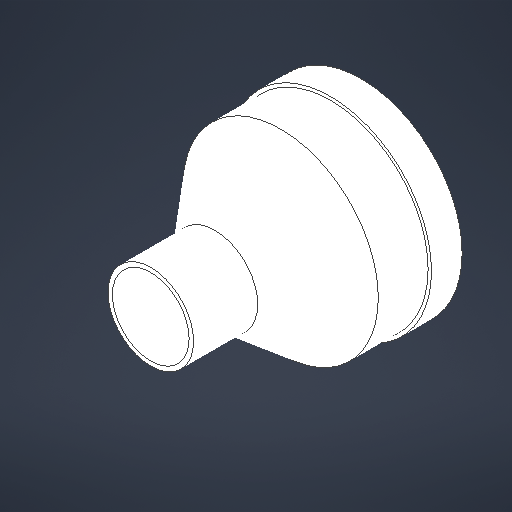
# Autodesk Inventor part: CAPSULA 2DA MITAD
Saved by Autodesk Inventor 2026.2 (Build 302298000, 298)
## iProperties
Created: 2025-12-31
Part Number: CAPSULA 2DA MITAD
Material: Genérico
Document SubType Name: Modeling
Designer: vicho
Density: 1 g/cm^3
Appearance: Valor por defecto
Author: vicho
Autodesk Inventor part; units mm, degrees
ref_plane "YZ Plane" through (0, 0, 0) normal (1, 0, 0) x (0, 1, 0)
ref_plane "XZ Plane" through (0, 0, 0) normal (0, 1, 0) x (-1, 0, 0)
sketch "Boceto1" plane through (0, 0, 0) normal (0, 0, 1) x (1, 0, 0)
  arc A0 (11.6645, -103.4622) -> (0, -112.3475) centre (12.4952, -116.6519) ccw construction
  line L0 (-152.4797, 0) -> (132.3175, 0) construction
  line L1 (0, 89.2085) -> (0, -112.3475) construction
  circle A1 centre (0, 0) radius 17.5
  dimension "d0" = 35
  constraints: 4 end point, 2 centre point, 2 point on circle, 2 point on line, 1 coincident, 1 horizontal, 1 vertical
  measures "d0" diameter of A1
extrude "Extrusión1" add sketch "Boceto1" along normal blind 30
ref_plane "Plano de trabajo1" through (0, 0, -30) normal (0, 0, 1) x (1, 0, 0)
sketch "Boceto2" plane through (0, 0, -30) normal (0, 0, 1) x (1, 0, 0)
  circle A0 centre (0, 0) radius 42.5
  dimension "d4" = 85
  constraints: 1 centre point, 1 coincident
  measures "d4" diameter of A0
loft "Solevación1" add profiles "Boceto2" section 2 edges at (-17.5, 0, 0)
ref_plane "Plano de trabajo2" through (0, 0, -55) normal (0, 0, 1) x (1, 0, 0)
sketch "Boceto3" plane through (0, 0, -55) normal (0, 0, 1) x (1, 0, 0)
  circle A0 centre (0, 0) radius 42.5
  dimension "d10" = 85
  constraints: 1 centre point, 1 coincident
  measures "d10" diameter of A0
loft "Solevación2" add profiles "Boceto3" section 2 edges at (-42.5, 0, -30)
shell "Vaciado1" thickness 2 outward yes removed faces 2 at (-10.6049, 7.3037, -55) at (4.865, -5.1831, 30)
ref_plane "Plano de trabajo3" through (0, 0, -52) normal (0, 0, 1) x (1, 0, 0)
sketch "Boceto4" plane through (0, 0, -52) normal (0, 0, 1) x (1, 0, 0)
  circle A0 centre (0, 0) radius 46.025
  dimension "d17" = 92.05
  constraints: 1 centre point, 1 coincident
  measures "d17" diameter of A0
extrude "Extrusión2" add sketch "Boceto4" against normal blind 14
sketch "Boceto5" plane through (0, 0, -66) normal (0, 0, -1) x (-1, 0, 0)
  circle A0 centre (0, 0) radius 44.525
  dimension "d20" = 89.05
  constraints: 1 centre point, 1 coincident
  measures "d20" diameter of A0
extrude "Extrusión3" cut sketch "Boceto5" against normal blind 12
sketch "Boceto6" plane through (0, 0, -54) normal (0, 0, -1) x (-1, 0, 0)
  circle A0 centre (0, 0) radius 42.5
  dimension "d23" = 85
  constraints: 1 centre point, 1 coincident
  measures "d23" diameter of A0
extrude "Extrusión4" cut sketch "Boceto6" against normal blind 12
